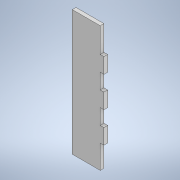
# Autodesk Inventor part: Side_2
Saved by Autodesk Inventor 2020 (Build 240168000, 168)
## iProperties
Created: 2020-12-28
Part Number: Side_2
Material: Generic
Document SubType Name: Modeling
Designer: solar
Density: 1 g/cm^3
Appearance: Default
Author: solar
Autodesk Inventor part; units mm, degrees
ref_plane "YZ Plane" through (0, 0, 0) normal (1, 0, 0) x (0, 1, 0)
ref_plane "XZ Plane" through (0, 0, 0) normal (0, 1, 0) x (-1, 0, 0)
ref_plane "XY Plane" through (0, 0, 0) normal (0, 0, 1) x (1, 0, 0)
sketch "Sketch1" plane through (0, 0, 0) normal (0, 0, 1) x (1, 0, 0)
  line L0 (-59, 61.875) -> (-59, 100)
  line L1 (-34, -100) -> (-54, -100)
  line L2 (-14, -12.375) -> (-8, -12.375)
  line L3 (-8, 37.125) -> (-14, 37.125)
  line L4 (-14, 61.875) -> (-8, 61.875)
  line L5 (-8, 12.375) -> (-14, 12.375)
  line L6 (-8, -37.125) -> (-14, -37.125)
  line L7 (-14, -61.875) -> (-8, -61.875)
  line L8 (-14, 61.875) -> (-14, 100)
  line L9 (-14, 37.125) -> (-14, 12.375)
  line L10 (-8, 37.125) -> (-8, 61.875)
  line L11 (-14, -12.375) -> (-14, -37.125)
  line L12 (-8, -61.875) -> (-8, -37.125)
  line L13 (-8, -12.375) -> (-8, 12.375)
  line L14 (-14, -61.875) -> (-14, -100)
  line L15 (-14, -100) -> (-59, -100)
  line L16 (-14, 100) -> (-14, 102)
  line L17 (-14, 102) -> (-59, 102)
  line L18 (-59, 102) -> (-59, 100)
  line L19 (-59, 61.875) -> (-59, -100)
  point P0 (-60, 61.875)
  point P1 (-60, 37.125)
  point P2 (-60, 12.375)
  point P3 (-60, -12.375)
  point P4 (-60, -37.125)
  point P5 (-60, -61.875)
  dimension "d23" = 45
  constraints: 40 end point, 2 collinear, 1 horizontal, 1 perpendicular, 1 vertical
  measures "d23" distance of L16.end L17.end
extrude "Extrusion1" add sketch "Sketch1" along normal blind 6
body "Solid1"
